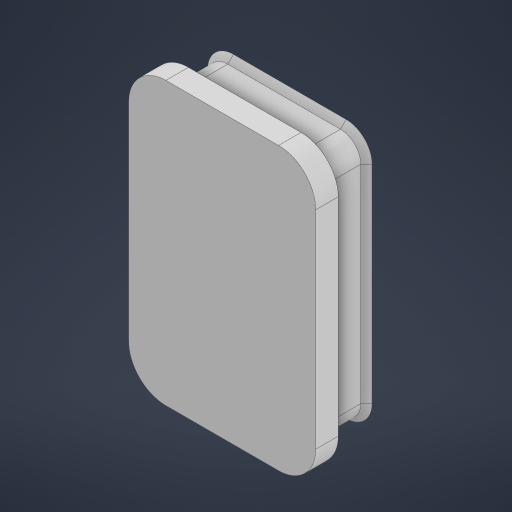
# Autodesk Inventor part: LilypadCover
Saved by Autodesk Inventor 2023 (Build 270158000, 158)
## iProperties
Created: 2022-07-23
Part Number: LilypadCover
Material: Generic
Document SubType Name: Modeling
Designer: jevan
Density: 1 g/cm^3
Appearance: Default
Author: jevan
Autodesk Inventor part; units mm, degrees
ref_plane "YZ Plane" through (0, 0, 0) normal (1, 0, 0) x (0, 1, 0)
ref_plane "XZ Plane" through (0, 0, 0) normal (0, 1, 0) x (-1, 0, 0)
ref_plane "XY Plane" through (0, 0, 0) normal (0, 0, 1) x (1, 0, 0)
sketch "Sketch1" plane through (0, 0, 0) normal (0, 0, 1) x (1, 0, 0)
  line L0 (-1, 0) -> (-6, 0)
  line L1 (-7, 1) -> (-7, 10.2)
  line L2 (-6, 11.2) -> (-1, 11.2)
  line L3 (0, 10.2) -> (0, 1)
  arc A0 (-7, 1) -> (-6, 0) centre (-6, 1) ccw
  arc A1 (-6, 11.2) -> (-7, 10.2) centre (-6, 10.2) ccw
  arc A2 (0, 10.2) -> (-1, 11.2) centre (-1, 10.2) ccw
  arc A3 (-1, 0) -> (0, 1) centre (-1, 1) ccw
  line L4 (-7.65, 10.2) -> (-7.65, 1)
  arc A4 (-7.65, 1) -> (-6, -0.65) centre (-6, 1) ccw
  line L5 (-6, -0.65) -> (-1, -0.65)
  arc A5 (-1, -0.65) -> (0.65, 1) centre (-1, 1) ccw
  line L6 (0.65, 1) -> (0.65, 10.2)
  arc A6 (0.65, 10.2) -> (-1, 11.85) centre (-1, 10.2) ccw
  line L7 (-1, 11.85) -> (-6, 11.85)
  arc A7 (-6, 11.85) -> (-7.65, 10.2) centre (-6, 10.2) ccw
  line L8 (-6.9, 10.2) -> (-6.9, 1)
  arc A8 (-6.9, 1) -> (-6, 0.1) centre (-6, 1) ccw
  line L9 (-6, 0.1) -> (-1, 0.1)
  arc A9 (-1, 0.1) -> (-0.1, 1) centre (-1, 1) ccw
  line L10 (-0.1, 1) -> (-0.1, 10.2)
  arc A10 (-0.1, 10.2) -> (-1, 11.1) centre (-1, 10.2) ccw
  line L11 (-1, 11.1) -> (-6, 11.1)
  arc A11 (-6, 11.1) -> (-6.9, 10.2) centre (-6, 10.2) ccw
  line L12 (-6.2, 1) -> (-6.2, 10.2)
  arc A12 (-6, 10.4) -> (-6.2, 10.2) centre (-6, 10.2) ccw
  line L13 (-6, 10.4) -> (-1, 10.4)
  arc A13 (-0.8, 10.2) -> (-1, 10.4) centre (-1, 10.2) ccw
  line L14 (-0.8, 10.2) -> (-0.8, 1)
  arc A14 (-1, 0.8) -> (-0.8, 1) centre (-1, 1) ccw
  line L15 (-1, 0.8) -> (-6, 0.8)
  arc A15 (-6.2, 1) -> (-6, 0.8) centre (-6, 1) ccw
  line L16 (-7.15, 10.2) -> (-7.15, 1)
  arc A16 (-7.15, 1) -> (-6, -0.15) centre (-6, 1) ccw
  line L17 (-6, -0.15) -> (-1, -0.15)
  arc A17 (-1, -0.15) -> (0.15, 1) centre (-1, 1) ccw
  line L18 (0.15, 1) -> (0.15, 10.2)
  arc A18 (0.15, 10.2) -> (-1, 11.35) centre (-1, 10.2) ccw
  line L19 (-1, 11.35) -> (-6, 11.35)
  arc A19 (-6, 11.35) -> (-7.15, 10.2) centre (-6, 10.2) ccw
  point P0 (0, 0)
  point P1 (-7, 11.2)
  point P2 (-7, 0)
  point P3 (0, 11.2)
  dimension "d0" = 7
  dimension "d1" = 11.2
  dimension "d2" = 1
  dimension "d3" = 0.65
  dimension "d6" = 0.1
  dimension "d9" = 0.7
  dimension "d10" = 0.15
  constraints: 40 end point, 40 point on circle, 20 centre point, 10 parallel, 8 point on line, 8 tangent, 5 perpendicular, 3 equal radius, 1 horizontal, 28 other
  measures "d0" distance of point (-7, 11.2) point (0, 11.2)
  measures "d1" distance of point (-7, 0) point (-7, 11.2)
  measures "d2" radius of A0
  measures "d3" distance between parallel lines of L1 L4
  measures "d6" distance between parallel lines of L1 L8
  measures "d9" distance between parallel lines of L8 L12
  measures "d10" distance between parallel lines of L1 L16
extrude "Extrusion1" add sketch "Sketch1" along normal blind 1 contours L0 A0 L1 A1 L2 A2 L3 A3 | A7 L7 A6 L6 A5 L5 A4 L4 | A11 L11 A10 L10 A9 L9 A8 L8 | L12 A12 L13 A13 L14 A14 L15 A15 | A19 L19 A18 L18 A17 L17 A16 L16
extrude "Extrusion2" add sketch "Sketch1" against normal blind 2 contours L0 A0 L1 A1 L2 A2 L3 A3 | A11 L11 A10 L10 A9 L9 A8 L8 | A19 L19 A18 L18 A17 L17 A16 L16
extrude "Extrusion3" cut sketch "Sketch1" against normal blind 1.75 contours L0 A0 L1 A1 L2 A2 L3 A3 | A19 L19 A18 L18 A17 L17 A16 L16
chamfer "Chamfer1" distance 0.25 distance2 0.25 8 edges at (-6.8132, 11.0132, -1.75) (-3.5, 11.35, -1.75) (-0.1868, 11.0132, -1.75) (0.15, 5.6, -1.75) (-0.1868, 0.1868, -1.75) (-3.5, -0.15, -1.75) (-6.8132, 0.1868, -1.75) (-7.15, 5.6, -1.75) measured on face at (-3.5, 11.25, -1.75) measured on face at (0.05, 5.6, -1.75) measured on face at (-3.5, -0.05, -1.75) measured on face at (-6.7425, 10.9425, -1.75) measured on face at (-7.05, 5.6, -1.75) measured on face at (-6.7425, 0.2575, -1.75) measured on face at (-0.2575, 10.9425, -1.75) measured on face at (-0.2575, 0.2575, -1.75)
body "Solid1"
